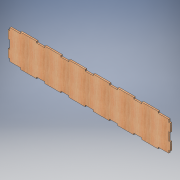
# Autodesk Inventor part: bottom
Saved by Autodesk Inventor 2016 (Build 200138000, 138)
## iProperties
Created: 2017-02-03
Part Number: bottom
Material: Wood (Birch)
Document SubType Name: Modeling
Designer: jwillauer
Density: 0.55 g/cm^3
Appearance: Birch - Natural Polished
Author: jwillauer
Autodesk Inventor part; units mm, degrees
ref_plane "YZ Plane" through (0, 0, 0) normal (1, 0, 0) x (0, 1, 0)
ref_plane "XZ Plane" through (0, 0, 0) normal (0, 1, 0) x (-1, 0, 0)
ref_plane "XY Plane" through (0, 0, 0) normal (0, 0, 1) x (1, 0, 0)
ref_plane "Work Plane1" through (0, 0, 19.05) normal (0, 0, 1) x (1, 0, 0)
sketch "Sketch2" plane through (0, 0, 19.05) normal (0, 0, 1) x (1, 0, 0)
  line L0 (1453.4656, 254.6366) -> (-578.5344, 254.6366) projected
  line L1 (-578.5344, 254.6366) -> (-559.4844, 254.6366)
  line L2 (-559.4844, -151.7634) -> (-578.5344, -151.7634)
  line L3 (-578.5344, -151.7634) -> (-578.5344, 254.6366)
  line L4 (1453.4656, -151.7634) -> (1453.4656, 254.6366) projected
  line L5 (-578.5344, -151.7634) -> (1453.4656, -151.7634) projected
  line L6 (1453.4656, 254.6366) -> (1434.4156, 254.6366)
  line L7 (1434.4156, -151.7634) -> (1453.4656, -151.7634)
  line L8 (1453.4656, -151.7634) -> (1453.4656, 254.6366)
  line L9 (-578.5344, 254.6366) -> (-578.5344, -151.7634) projected
  line L10 (-559.4844, 254.6366) -> (-559.4844, 203.8366)
  line L11 (-578.5344, 203.8366) -> (-559.4844, 203.8366)
  line L12 (1434.4156, 203.8366) -> (1453.4656, 203.8366)
  line L13 (-578.5344, 102.2366) -> (-559.4844, 102.2366)
  line L14 (1434.4156, 102.2366) -> (1453.4656, 102.2366)
  line L15 (-578.5344, 0.6366) -> (-559.4844, 0.6366)
  line L16 (1434.4156, 0.6366) -> (1453.4656, 0.6366)
  line L17 (-578.5344, -100.9634) -> (-559.4844, -100.9634)
  line L18 (1434.4156, -100.9634) -> (1453.4656, -100.9634)
  line L19 (-559.4844, 102.2366) -> (-559.4844, 0.6366)
  line L20 (-559.4844, -100.9634) -> (-559.4844, -151.7634)
  line L21 (1434.4156, 254.6366) -> (1434.4156, 203.8366)
  line L22 (1434.4156, 102.2366) -> (1434.4156, 0.6366)
  line L23 (1434.4156, -100.9634) -> (1434.4156, -151.7634)
  line L24 (-578.5344, 254.6366) -> (-559.4844, 254.6366)
  line L25 (-559.4844, 254.6366) -> (-559.4844, 203.8366)
  line L26 (-559.4844, 203.8366) -> (-578.5344, 203.8366)
  line L27 (-578.5344, 203.8366) -> (-578.5344, 254.6366)
  line L28 (-578.5344, 102.2366) -> (-559.4844, 102.2366)
  line L29 (-559.4844, 102.2366) -> (-559.4844, 0.6366)
  line L30 (-559.4844, 0.6366) -> (-578.5344, 0.6366)
  line L31 (-578.5344, 0.6366) -> (-578.5344, 102.2366)
  line L32 (-578.5344, -100.9634) -> (-559.4844, -100.9634)
  line L33 (-559.4844, -100.9634) -> (-559.4844, -151.7634)
  line L34 (-559.4844, -151.7634) -> (-578.5344, -151.7634)
  line L35 (-578.5344, -151.7634) -> (-578.5344, -100.9634)
  line L36 (1453.4656, 254.6366) -> (1434.4156, 254.6366)
  line L37 (1434.4156, 254.6366) -> (1434.4156, 203.8366)
  line L38 (1434.4156, 203.8366) -> (1453.4656, 203.8366)
  line L39 (1453.4656, 203.8366) -> (1453.4656, 254.6366)
  line L40 (1453.4656, 102.2366) -> (1434.4156, 102.2366)
  line L41 (1434.4156, 102.2366) -> (1434.4156, 0.6366)
  line L42 (1434.4156, 0.6366) -> (1453.4656, 0.6366)
  line L43 (1453.4656, 0.6366) -> (1453.4656, 102.2366)
  line L44 (1453.4656, -100.9634) -> (1434.4156, -100.9634)
  line L45 (1434.4156, -100.9634) -> (1434.4156, -151.7634)
  line L46 (1434.4156, -151.7634) -> (1453.4656, -151.7634)
  line L47 (1453.4656, -151.7634) -> (1453.4656, -100.9634)
  point P0 (0, 0)
  constraints: 88 end point, 20 parallel, 14 horizontal, 12 perpendicular, 9 point on line
extrude "Extrusion2" add sketch "Sketch2" along normal blind 19.05 contours L21 L12 L4 L14 L22 L16 L18 L23 L5 L20 L17 L3 L15 L19 L13 L11 L10 L0
sketch "Sketch3" plane through (0, 0, 38.1) normal (0, 0, 1) x (1, 0, 0)
  line L0 (1434.4156, 254.6366) -> (-559.4844, 254.6366) projected
  line L1 (1453.4656, 102.2366) -> (1453.4656, 203.8366) projected
  line L2 (-559.4844, -151.7634) -> (1434.4156, -151.7634) projected
  line L3 (-559.4844, 254.6366) -> (-426.1344, 254.6366)
  line L4 (-559.4844, 235.5866) -> (-426.1344, 235.5866)
  line L5 (-222.9344, 254.6366) -> (-121.3344, 254.6366)
  line L6 (-222.9344, 235.5866) -> (-121.3344, 235.5866)
  line L7 (81.8656, 254.6366) -> (183.4656, 254.6366)
  line L8 (81.8656, 235.5866) -> (183.4656, 235.5866)
  line L9 (386.6656, 254.6366) -> (488.2656, 254.6366)
  line L10 (386.6656, 235.5866) -> (488.2656, 235.5866)
  line L11 (691.4656, 254.6366) -> (793.0656, 254.6366)
  line L12 (691.4656, 235.5866) -> (793.0656, 235.5866)
  line L13 (996.2656, 254.6366) -> (1097.8656, 254.6366)
  line L14 (1301.0656, 254.6366) -> (1434.4156, 254.6366)
  line L15 (996.2656, 235.5866) -> (1097.8656, 235.5866)
  line L16 (1301.0656, 235.5866) -> (1434.4156, 235.5866)
  line L17 (1301.0656, 254.6366) -> (1301.0656, 235.5866)
  line L18 (1301.0656, -132.7134) -> (1301.0656, -151.7634)
  line L19 (1097.8656, 254.6366) -> (1097.8656, 235.5866)
  line L20 (1097.8656, -132.7134) -> (1097.8656, -151.7634)
  line L21 (996.2656, 254.6366) -> (996.2656, 235.5866)
  line L22 (996.2656, -132.7134) -> (996.2656, -156.6063)
  line L23 (793.0656, 254.6366) -> (793.0656, 235.5866)
  line L24 (793.0656, -132.7134) -> (793.0656, -151.7634)
  line L25 (691.4656, 254.6366) -> (691.4656, 235.5866)
  line L26 (691.4656, -132.7134) -> (691.4656, -151.7634)
  line L27 (488.2656, 254.6366) -> (488.2656, 235.5866)
  line L28 (488.2656, -132.7134) -> (488.2656, -151.7634)
  line L29 (386.6656, 254.6366) -> (386.6656, 235.5866)
  line L30 (386.6656, -132.7134) -> (386.6656, -151.7634)
  line L31 (183.4656, 254.6366) -> (183.4656, 235.5866)
  line L32 (183.4656, -132.7134) -> (183.4656, -151.7634)
  line L33 (81.8656, 254.6366) -> (81.8656, 235.5866)
  line L34 (81.8656, -132.7134) -> (81.8656, -151.7634)
  line L35 (-121.3344, 254.6366) -> (-121.3344, 235.5866)
  line L36 (-121.3344, -132.7134) -> (-121.3344, -156.6063)
  line L37 (-222.9344, 254.6366) -> (-222.9344, 235.5866)
  line L38 (-222.9344, -132.7134) -> (-222.9344, -151.7634)
  line L39 (-426.1344, 254.6366) -> (-426.1344, 235.5866)
  line L40 (-426.1344, -132.7134) -> (-426.1344, -151.7634)
  line L41 (-426.1344, -132.7134) -> (-559.4844, -132.7134)
  line L42 (-559.4844, -132.7134) -> (-426.1344, -132.7134)
  line L43 (-426.1344, -151.7634) -> (-559.4844, -151.7634)
  line L44 (-121.3344, -132.7134) -> (-222.9344, -132.7134)
  line L45 (-121.3344, -151.7634) -> (-222.9344, -151.7634)
  line L46 (-222.9344, -132.7134) -> (-121.3344, -132.7134)
  line L47 (183.4656, -151.7634) -> (81.8656, -151.7634)
  line L48 (183.4656, -132.7134) -> (81.8656, -132.7134)
  line L49 (81.8656, -132.7134) -> (183.4656, -132.7134)
  line L50 (488.2656, -132.7134) -> (386.6656, -132.7134)
  line L51 (488.2656, -151.7634) -> (386.6656, -151.7634)
  line L52 (386.6656, -132.7134) -> (488.2656, -132.7134)
  line L53 (793.0656, -132.7134) -> (691.4656, -132.7134)
  line L54 (793.0656, -151.7634) -> (691.4656, -151.7634)
  line L55 (691.4656, -132.7134) -> (793.0656, -132.7134)
  line L56 (1434.4156, -132.7134) -> (1301.0656, -132.7134)
  line L57 (1097.8656, -132.7134) -> (996.2656, -132.7134)
  line L58 (1434.4156, -151.7634) -> (1301.0656, -151.7634)
  line L59 (1097.8656, -151.7634) -> (996.2656, -151.7634)
  line L60 (996.2656, -132.7134) -> (1097.8656, -132.7134)
  line L61 (1301.0656, -132.7134) -> (1434.4156, -132.7134)
  line L62 (1434.4156, 254.6366) -> (1434.4156, 235.5866)
  line L63 (1434.4156, -132.7134) -> (1434.4156, -151.7634)
  line L64 (-559.4844, 254.6366) -> (-559.4844, 235.5866)
  line L65 (-559.4844, -132.7134) -> (-559.4844, -151.7634)
  point P0 (0, 0)
  point P1 (1453.4656, -132.7134)
  point P2 (1545.8427, 235.5866)
  point P3 (874.9313, 0)
  constraints: 126 end point, 38 perpendicular, 14 point on line, 7 horizontal, 7 parallel
extrude "Extrusion3" cut sketch "Sketch3" against normal blind 19.05
body "Solid2"
